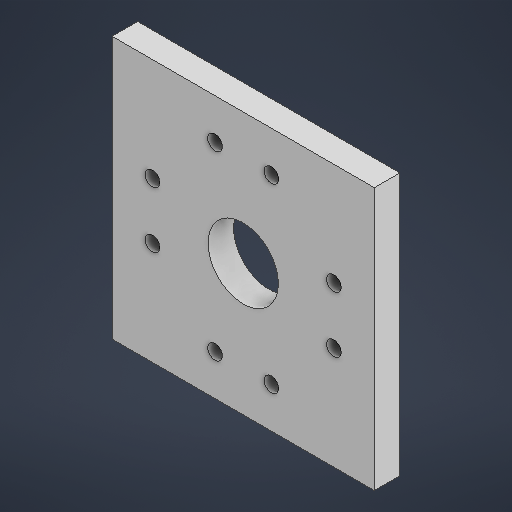
# Autodesk Inventor part: servo_attachment
Saved by Autodesk Inventor 2026 (Build 300175000, 175)
## iProperties
Created: 2025-07-02
Part Number: servo_attachment
Material: Generic
Document SubType Name: Modeling
Designer: user
Density: 1 g/cm^3
Appearance: Default
Author: user
Autodesk Inventor part; units mm, degrees
ref_plane "YZ Plane" through (0, 0, 0) normal (1, 0, 0) x (0, 1, 0)
ref_plane "XZ Plane" through (0, 0, 0) normal (0, 1, 0) x (-1, 0, 0)
ref_plane "XY Plane" through (0, 0, 0) normal (0, 0, 1) x (1, 0, 0)
sketch "Sketch1" plane through (0, 0, 0) normal (0, 0, 1) x (1, 0, 0)
  line L0 (-20.5, -20.5) -> (20.5, -20.5)
  line L1 (20.5, -20.5) -> (20.5, 20.5)
  line L2 (20.5, 20.5) -> (-20.5, 20.5)
  line L3 (-20.5, 20.5) -> (-20.5, -20.5)
  line L4 (-20.5, -20.5) -> (20.5, 20.5) construction
  line L5 (20.5, -20.5) -> (-20.5, 20.5) construction
  point P0 (0, 0)
  dimension "d0" = 41
  dimension "d1" = 41
  constraints: 12 end point, 2 midpoint, 2 parallel, 1 horizontal, 1 perpendicular
  measures "d0" distance of L2.end L1.end
  measures "d1" distance of L1.end L0.end
extrude "Extrusion1" add sketch "Sketch1" along normal blind 4
sketch "Sketch2" plane through (0, 0, 4) normal (0, 0, 1) x (1, 0, 0)
  circle A0 centre (0, 0) radius 5.5
  dimension "d4" = 11
  constraints: 1 centre point, 1 coincident
  measures "d4" diameter of A0
extrude "Extrusion2" cut sketch "Sketch2" against normal blind 4
sketch "Sketch3" plane through (0, 0, 4) normal (0, 0, 1) x (1, 0, 0)
  circle A0 centre (0, 0) radius 5.5 projected
  circle A1 centre (0, 0) radius 6.45
  circle A2 centre (-18.375, 0) radius 2.125
  circle A3 centre (18.375, 0) radius 2.125
  line L0 (-18.721, 2.0966) -> (-4.7075, 4.4093)
  line L1 (-18.7594, -2.0899) -> (-4.3799, -4.7348)
  line L2 (18.7217, 2.0965) -> (4.702, 4.4152)
  line L3 (18.7594, -2.0899) -> (4.3799, -4.7348)
  line L4 (0, 0) -> (18.375, 0)
  line L5 (0, 0) -> (-18.375, 0)
  circle A4 centre (-14.175, -4.4) radius 1.15
  circle A5 centre (14.175, 4.4) radius 1.15
  dimension "d7" = 12.9
  dimension "d8" = 4.25
  dimension "d9" = 4.25
  dimension "d10" = 9.15
  dimension "d11" = 9.15
  dimension "d12" = 41
  dimension "d13" = 18.375
  dimension "d14" = 2.3
  dimension "d15" = 4.4
  dimension "d16" = 4.2
  dimension "d17" = 2.3
  dimension "d18" = 4.4
  dimension "d19" = 4.2
  constraints: 12 end point, 8 point on circle, 5 centre point, 4 tangent, 2 coincident, 2 horizontal
  measures "d7" diameter of A1
  measures "d8" diameter of A2
  measures "d9" diameter of A3
  measures "d10" distance of L1.end L0.end
  measures "d11" vertical distance of L3.end L2.end
  measures "d13" distance of L5.start L5.end
  measures "d14" diameter of A4
  measures "d15" distance from line of L5 A4.centre
  measures "d16" horizontal distance of L5.end A4.centre
  measures "d17" diameter of A5
  measures "d18" distance from line of L4 A5.centre
  measures "d19" horizontal distance of A5.centre L4.end
extrude "Extrusion3" cut sketch "Sketch3" against normal blind 4 contours A4 | A5
mirror "Mirror1" about plane through (0, 0, 0) normal (0, 1, 0) of "Extrusion3"
pattern_circular "Circular Pattern1" count 4 over 360 about axis through (0, 0, 4) along (0, 0, -1) of "Extrusion3", "Mirror1"
body "Solid1"
